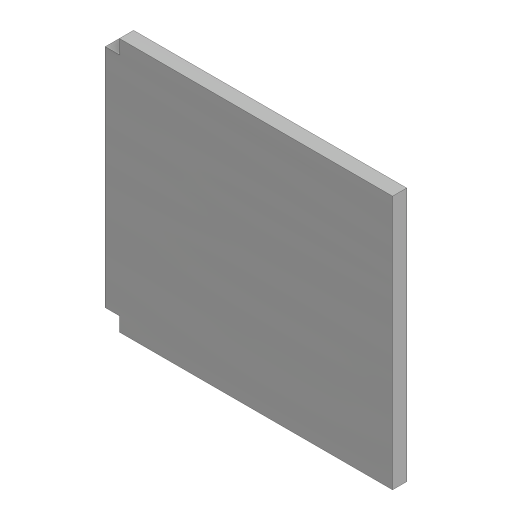
# Autodesk Inventor part: II Bodenplatte kurz
Saved by Autodesk Inventor 2023 (Build 270158000, 158)
## iProperties
Created: 2022-09-26
Part Number: II Bodenplatte kurz
Material: PVC, hart
Document SubType Name: Modeling
Designer: musati
Density: 1.29 g/cm^3
Appearance: Light Gray
Author: musati
Autodesk Inventor part; units mm, degrees
ref_plane "YZ Plane" through (0, 0, 0) normal (1, 0, 0) x (0, 1, 0)
ref_plane "XZ Plane" through (0, 0, 0) normal (0, 1, 0) x (-1, 0, 0)
ref_plane "XY Plane" through (0, 0, 0) normal (0, 0, 1) x (1, 0, 0)
sketch "Skizze1" plane through (0, 0, 0) normal (0, 0, 1) x (1, 0, 0)
  line L0 (-85.4, 0) -> (85.4, 0) projected
  line L1 (0, -75.6) -> (0, 75.6) projected
  line L2 (-61, -54) -> (61, -54)
  line L3 (61, -54) -> (61, 54)
  line L4 (61, 54) -> (-61, 54)
  line L5 (-61, 54) -> (-61, -54)
  line L6 (-61, -54) -> (61, 54) construction
  line L7 (61, -54) -> (-61, 54) construction
  point P0 (0, 0)
  dimension "d0" = 122
  dimension "d1" = 108
  constraints: 12 end point, 2 midpoint, 2 parallel, 1 horizontal, 1 perpendicular
  measures "d0" distance of L4.end L3.end
  measures "d1" distance of L3.end L2.end
extrude "Extrusion1" add sketch "Skizze1" against normal blind 6
sketch "Skizze2" plane through (0, 0, 0) normal (0, 0, 1) x (1, 0, 0)
  line L0 (-61, -54) -> (61, -54) projected
  line L1 (61, -54) -> (61, 54) projected
  line L2 (61, 54) -> (-61, 54) projected
  line L3 (-61, 54) -> (-61, -54) projected
  line L4 (-85.4, 0) -> (85.4, 0) projected
  line L5 (0, -75.6) -> (0, 75.6) projected
  line L6 (-61, 54) -> (-55, 54)
  line L7 (-55, 54) -> (-55, 48)
  line L8 (-55, 48) -> (-61, 48)
  line L9 (-61, 48) -> (-61, 54)
  line L10 (61, -54) -> (-61, -54) projected
  line L11 (-61, -54) -> (-55, -54)
  line L12 (-55, -54) -> (-55, -48)
  line L13 (-55, -48) -> (-61, -48)
  line L14 (-61, -48) -> (-61, -54)
  point P0 (0, 0)
  dimension "d4" = 6
  dimension "d5" = 6
  dimension "d6" = 6
  dimension "d7" = 6
  constraints: 16 end point, 4 parallel, 2 horizontal, 2 perpendicular
  measures "d4" distance of L7.end L8.end
  measures "d5" distance of L6.end L7.end
  measures "d6" distance of L13.end L12.end
  measures "d7" distance of L12.end L11.end
extrude "Extrusion2" cut sketch "Skizze2" against normal blind 6 contours L3 L13 L12 L0 | L3 L2 L7 L8
